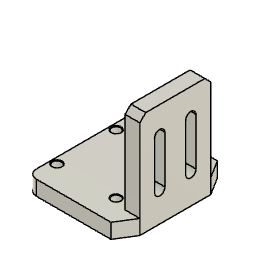
Magneto+Eddy+Mount (Autodesk Fusion 360 design; units mm, degrees)
Autodesk Fusion 360 part; units mm, degrees
note: some values were not read from the file. Chosen so that the rebuilt part matches the saved one: which face or edge a step refers to.
sketch "Skizze1" plane through (0, 0, 0) normal (0, 0, 1) x (1, 0, 0)
  circle A0 centre (0, 20) radius 1.5
  circle A1 centre (20, 20) radius 1.5
  circle A2 centre (0, 0) radius 1.5
  circle A3 centre (20, 0) radius 1.5
  line L0 (0, 30) -> (30, 30)
  line L1 (30, 30) -> (30, -10)
  line L2 (30, -10) -> (0, -10)
  line L3 (0, 30) -> (-2, 30)
  line L4 (0, -10) -> (-2, -10)
  line L5 (-2, -10) -> (-2, 30)
  line L6 (30, 30) -> (25, 30)
  line L7 (25, 30) -> (25, -10)
  line L8 (25, -10) -> (30, -10)
  line L9 (30, -10) -> (30, 30)
  dimension "d1" = 20
  dimension "d2" = 20
  dimension "d3" = 3
  dimension "d4" = 3
  dimension "d5" = 3
  dimension "d6" = 3
  dimension "d10" = 10
  dimension "d11" = 10
  dimension "d13" = 2
  dimension "d15" = 2
  constraint coincident A2.centre origin
  constraint horizontal L0
  constraint vertical L1
  constraint horizontal L2
  constraint perpendicular L3 L5
  constraint horizontal L6
  constraint vertical L7
  constraint horizontal L8
  constraint vertical L9
  constraint coincident L2 L7.end
  measures "d1" distance of A2.centre A3.centre
  measures "d2" distance of A2.centre A0.centre
  measures "d3" diameter of A0
  measures "d4" diameter of A1
  measures "d5" diameter of A2
  measures "d6" diameter of A3
  measures "d10" distance of A2.centre L2.end
  measures "d11" distance of A0.centre L0.start
  measures "d13" distance of L0.start L3.end
  measures "d15" distance of L2.end L4.end
extrude "Extrusion1" add sketch "Skizze1" along normal blind 5
extrude "Extrusion2" add sketch "Skizze1" along normal blind 35 contours L0 L1 L2 L6 L7 L8 L9
sketch "Skizze2" plane through (25, 0, 0) normal (-1, 0, 0) x (0, -1, 0)
  line L0 (-30, 5) -> (10, 5)
  line L1 (10, 5) -> (10, 35)
  line L2 (-30, 35) -> (-30, 5)
  line L3 (-13.5, 26) -> (-13.5, 10)
  line L4 (-3, 26) -> (-3, 10)
  line L5 (-17, 26) -> (-17, 10)
  line L6 (-6.5, 10) -> (-6.5, 26)
  arc A0 (-13.5, 26) -> (-17, 26) centre (-15.25, 26) ccw
  arc A1 (-3, 26) -> (-6.5, 26) centre (-4.75, 26) ccw
  arc A2 (-6.5, 10) -> (-3, 10) centre (-4.75, 10) ccw
  arc A3 (-17, 10) -> (-13.5, 10) centre (-15.25, 10) ccw
  dimension "d21" = 10.5
  dimension "d22" = 3.5
  dimension "d23" = 3.5
  dimension "d24" = 10.5
  dimension "d25" = 3.5
  dimension "d26" = 3.5
  constraint tangent L3 A3
  constraint tangent L4 A2
  constraint tangent L5 A3
  constraint tangent L6 A1
  constraint parallel L5 L6
  measures "d21" distance of A1.centre A0.centre
  measures "d22" diameter of A1
  measures "d23" diameter of A0
  measures "d24" distance of A3.centre A2.centre
  measures "d25" diameter of A2
  measures "d26" diameter of A3
extrude "Extrusion3" cut sketch "Skizze2" against normal blind 32
sketch "Skizze3" plane through (0, 0, 5) normal (0, 0, 1) x (-1, 0, 0)
  line L0 (-25, 10) -> (-25, -30)
  line L1 (-25, -30) -> (2, -30)
  line L2 (2, -30) -> (2, 10)
  line L3 (2, 10) -> (-25, 10)
  circle A0 centre (0, 0) radius 1.5
  circle A1 centre (-20, 0) radius 1.5
  circle A2 centre (0, -20) radius 1.5
  circle A3 centre (-20, -20) radius 1.5
  line L4 (-19, -17.5) -> (-25, -17.5)
  line L5 (-19, -2.5) -> (-25, -2.5)
  line L6 (-19, -17.5) -> (-19, -2.5)
extrude "Extrusion4" cut sketch "Skizze3" against normal blind 13 contours L0 L4 L5 L6
chamfer "Fase1" distance 10 angle 45 2 edges at (27.5, -10, 35) (27.5, 30, 35)
sketch "Skizze4" plane through (25, 0, 0) normal (-1, 0, 0) x (0, -1, 0)
  line L0 (-17, 10) -> (-17, 26)
  arc A0 (-13.5, 26) -> (-17, 26) centre (-15.25, 26) ccw
  line L1 (-13.5, 26) -> (-13.5, 10)
  arc A1 (-17, 10) -> (-13.5, 10) centre (-15.25, 10) ccw
  line L2 (-6.5, 10) -> (-6.5, 26)
  arc A2 (-3, 26) -> (-6.5, 26) centre (-4.75, 26) ccw
  line L3 (-3, 26) -> (-3, 10)
  arc A3 (-6.5, 10) -> (-3, 10) centre (-4.75, 10) ccw
  line L4 (-20, 35) -> (-30, 25)
  line L5 (-30, 25) -> (-30, 5)
  line L6 (-30, 5) -> (-17.5, 5)
  line L7 (-17.5, 5) -> (-17.5, 0)
  line L8 (-17.5, 0) -> (-2.5, 0)
  line L9 (-2.5, 0) -> (-2.5, 5)
  line L10 (-2.5, 5) -> (10, 5)
  line L11 (10, 5) -> (10, 25)
  line L12 (10, 25) -> (0, 35)
  line L13 (0, 35) -> (-20, 35)
  arc A4 (-2.5, 5) -> (-17.5, 5) centre (-10, -5) ccw
  constraint coincident L9.end L10.start
  constraint coincident L6.end L7.start
extrude "Extrusion5" cut sketch "Skizze4" against normal blind 6.5 contours L7 L8 L9 A4
fillet "Abrundung1" radius 3 2 edges at (19, 17.5, 2.5) (19, 2.5, 2.5)
fillet "Abrundung2" radius 2 2 edges at (-2, 30, 2.5) (-2, -10, 2.5)
sketch "Skizze5" plane through (0, -10, 0) normal (0, -1, 0) x (1, 0, 0)
  line L0 (0, 5) -> (0, 0)
  line L1 (0, 0) -> (30, 0)
  line L2 (30, 0) -> (30, 25)
  line L3 (30, 25) -> (25, 25)
  line L4 (25, 25) -> (25, 5)
  line L5 (25, 5) -> (0, 5)
  line L6 (30, 25) -> (25, 25)
  line L7 (25, 25) -> (25, 0)
  line L8 (25, 0) -> (30, 0)
  line L9 (30, 0) -> (30, 25)
  line L10 (25, 25, -40) -> (30, 25, -40)
  line L11 (30, 25, -40) -> (30, 0, -40)
  line L12 (30, 0, -40) -> (25, 0, -40)
  line L13 (25, 0, -40) -> (25, 25, -40)
  point P0 (25, 25)
  point P1 (30, 0)
  constraint horizontal L6
  constraint vertical L7
  constraint horizontal L8
  constraint vertical L9
  constraint coincident L2.end L3.start
  constraint coincident P1 L1.end
  constraint coincident P0 L3.end
sketch "Skizze5 (curves -40 mm off its plane)" plane through (0, 30, 0) normal (0, -1, 0) x (1, 0, 0)
  line L0 (25, 25) -> (30, 25)
  line L1 (30, 25) -> (30, 0)
  line L2 (30, 0) -> (25, 0)
  line L3 (25, 0) -> (25, 25)
extrude "Extrusion6" cut sketch "Skizze5 (curves -40 mm off its plane)" along normal blind 10
extrude "Extrusion7" cut sketch "Skizze5" against normal blind 10 contours L1 L2 L3 L4 L6 L7 L8 L9
extrude "Extrusion8" add 1 faces at (28.3333, 20, 10) along direction (0, 1, 0) blind 2
extrude "Extrusion9" add 1 faces at (28.3333, 0, 10) along direction (0, -1, 0) blind 2
extrude "Extrusion10" cut 1 faces at (28.3333, -7.3333, 25) along direction (0, 0, 1) blind 15
extrude "Extrusion11" cut 1 faces at (26.6667, 27.3333, 25) along direction (0, 0, 1) blind 15
sketch "Skizze6" plane through (0, 0, 5) normal (0, 0, 1) x (-1, 0, 0)
  arc A0 (2, 8) -> (0, 10) centre (0, 8) ccw
  line L0 (0, 10) -> (-25, 10)
  line L1 (-25, 10) -> (-25, 2)
  line L2 (-25, 2) -> (-25, -2.5)
  line L3 (-25, -2.5) -> (-22, -2.5)
  arc A1 (-19, -5.5) -> (-22, -2.5) centre (-22, -5.5) ccw
  line L4 (-19, -5.5) -> (-19, -14.5)
  arc A2 (-22, -17.5) -> (-19, -14.5) centre (-22, -14.5) ccw
  line L5 (-22, -17.5) -> (-25, -17.5)
  line L6 (-25, -17.5) -> (-25, -22)
  line L7 (-25, -22) -> (-25, -30)
  line L8 (-25, -30) -> (0, -30)
  arc A3 (0, -30) -> (2, -28) centre (0, -28) ccw
  line L9 (2, -28) -> (2, 8)
  circle A4 centre (-20, -20) radius 1.5
  circle A5 centre (0, -20) radius 1.5
  circle A6 centre (-20, 0) radius 1.5
  circle A7 centre (0, 0) radius 1.5
  line L10 (-30, 2, -5) -> (-25, 10, -5)
  line L11 (-25, 10, -5) -> (-25, 2, -5)
  line L12 (-25, 2, -5) -> (-30, 2, -5)
  line L13 (-30, -22, -5) -> (-25, -30, -5)
  line L14 (-25, -30, -5) -> (-25, -22, -5)
  line L15 (-25, -22, -5) -> (-30, -22, -5)
  point P0 (-30, 2)
  point P1 (-25, 10)
  point P2 (-25, 2)
  point P3 (-30, 2)
  point P4 (-30, -22)
  point P5 (-25, -30)
  point P6 (-25, -22)
  point P7 (-30, -22)
  constraint coincident P3 P0
  constraint coincident P1 L0.end
  constraint coincident P2 L1.end
  constraint coincident P7 P4
  constraint coincident P5 L7.end
  constraint coincident P6 L6.end
sketch "Skizze6 (curves -5 mm off its plane)" plane through (0, 0, 0) normal (0, 0, 1) x (-1, 0, 0)
  line L0 (-30, 2) -> (-25, 10)
  line L1 (-25, 10) -> (-25, 2)
  line L2 (-25, 2) -> (-30, 2)
  line L3 (-30, -22) -> (-25, -30)
  line L4 (-25, -30) -> (-25, -22)
  line L5 (-25, -22) -> (-30, -22)
extrude "Extrusion12" add sketch "Skizze6 (curves -5 mm off its plane)" along normal blind 5 contours L3 L4 L5
extrude "Extrusion13" add sketch "Skizze6 (curves -5 mm off its plane)" along normal blind 5 contours L0 L1 L2
chamfer "Fase2" distance 0.2 angle 45 4 edges at (18.6015, 20.5424, 5) (-1.3985, 20.5424, 5) (18.6015, 0.5424, 5) (-1.3985, 0.5424, 5)
extrude "Extrusion14" cut 1 faces at (16.6667, -10, 3.3333) along direction (0, 1, 0) blind 2
extrude "Extrusion15" cut 1 faces at (8.3333, 30, 3.3333) along direction (0, -1, 0) blind 2
extrude "Extrusion16" cut 1 faces at (25, 29.3333, 1.6667) along direction (1, 0, 0) blind 7
extrude "Extrusion17" cut 1 faces at (25, -9.3333, 3.3333) along direction (1, 0, 0) blind 7
extrude "Extrusion18" cut 1 faces at (0, 29.3333, 1.6667) along direction (-1, 0, 0) blind 7
extrude "Extrusion19" cut 1 faces at (0, -8.6667, 3.3333) along direction (-1, 0, 0) blind 9
fillet "Abrundung3" radius 3 1 edges at (-2, -8, 2.5)
fillet "Abrundung3" radius 3 1 edges at (-2, 28, 2.5)
extrude "Extrusion20" add 1 faces at (19, 11.5, 3.3333) along direction (1, 0, 0) blind 11
extrude "Extrusion21" add 1 faces at (22.6667, 14.5, 3.3333) along direction (0, 1, 0) blind 4
extrude "Extrusion22" add 1 faces at (22.6667, 5.5, 3.3333) along direction (0, -1, 0) blind 4
sketch "Skizze7" plane through (30, 0, 0) normal (1, 0, 0) x (0, 1, 0)
  line L0 (-2, 0) -> (22, 0)
  line L1 (22, 0) -> (22, 5)
  line L2 (22, 5) -> (22, 33)
  line L3 (22, 33) -> (20, 35)
  line L4 (20, 35) -> (0, 35)
  line L5 (0, 35) -> (-2, 33)
  line L6 (-2, 33) -> (-2, 5)
  line L7 (-2, 5) -> (-2, 0)
  line L8 (17.5, 5) -> (2.5, 5)
  arc A0 (17.5, 5) -> (2.5, 5) centre (10, -5) ccw
  line L9 (17, 26) -> (17, 10)
  arc A1 (13.5, 10) -> (17, 10) centre (15.25, 10) ccw
  line L10 (13.5, 10) -> (13.5, 26)
  arc A2 (17, 26) -> (13.5, 26) centre (15.25, 26) ccw
  line L11 (6.5, 26) -> (6.5, 10)
  arc A3 (3, 10) -> (6.5, 10) centre (4.75, 10) ccw
  line L12 (3, 10) -> (3, 26)
  arc A4 (6.5, 26) -> (3, 26) centre (4.75, 26) ccw
  line L13 (2, 8) -> (18, 8)
  line L14 (18, 8) -> (18, 3)
  line L15 (18, 3) -> (2, 3)
  line L16 (2, 3) -> (2, 8)
  constraint horizontal L13
  constraint vertical L14
  constraint horizontal L15
  constraint vertical L16
extrude "Extrusion23" add sketch "Skizze7" against normal blind 5 contours L8 A0 | L13 L14 L15 L16
